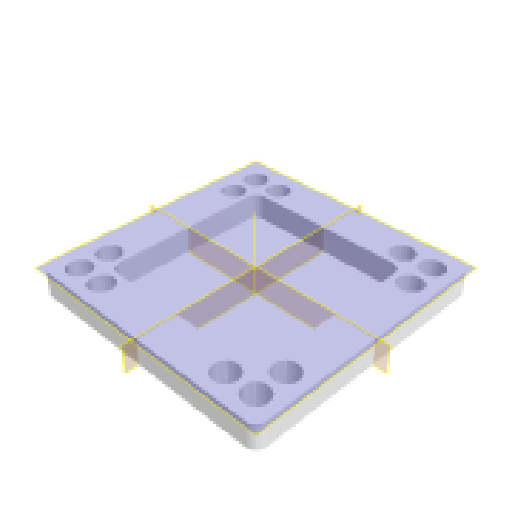
# Autodesk Inventor part: 10_Base_v4
Saved by Autodesk Inventor 2025.1 (Build 291241020, 241B)
## iProperties
Created: 2024-08-19
Part Number: 10_Base_v4
Material: Generisch
Document SubType Name: Modeling
Designer: diederichbenedict
Density: 1 g/cm^3
Appearance: Smooth - White
Author: diederichbenedict
Autodesk Inventor part; units mm, degrees
ref_plane "YZ Plane" through (0, 0, 0) normal (1, 0, 0) x (0, 1, 0)
ref_plane "XZ Plane" through (0, 0, 0) normal (0, 1, 0) x (-1, 0, 0)
ref_plane "XY Plane" through (0, 0, 0) normal (0, 0, 1) x (1, 0, 0)
ref_plane "Arbeitsebene1" through (21.5439, 0, 2.0695) normal (0, 0, -1) x (-1, 0, 0)
sketch "Skizze1" plane through (21.5439, 0, 2.0695) normal (0, 0, -1) x (-1, 0, 0)
  line L0 (-25, -25) -> (25, -25)
  line L1 (25, -25) -> (25, 25)
  line L2 (25, 25) -> (-25, 25)
  line L3 (-25, 25) -> (-25, -25)
  line L4 (-25, -25) -> (25, 25) construction
  line L5 (25, -25) -> (-25, 25) construction
  line L6 (-17, -17) -> (17, -17)
  line L7 (17, -17) -> (17, 17)
  line L8 (17, 17) -> (-17, 17)
  line L9 (-17, 17) -> (-17, -17)
  line L10 (-17, -17) -> (17, 17) construction
  line L11 (17, -17) -> (-17, 17) construction
  point P0 (21.5439, 0)
  point P1 (0, 0)
  point P2 (0, 0)
  dimension "d0" = 50
  dimension "d1" = 50
  dimension "d2" = 34
  dimension "d3" = 34
  constraints: 24 end point, 5 midpoint, 4 parallel, 2 horizontal, 2 perpendicular
  measures "d0" distance of L2.end L1.end
  measures "d1" distance of L1.end L0.end
  measures "d2" distance of L8.end L7.end
  measures "d3" distance of L7.end L6.end
extrude "Extrusion1" add sketch "Skizze1" along normal blind 5
sketch "Skizze2" plane through (21.5439, 0, -2.9305) normal (0, 0, -1) x (-1, 0, 0)
  line L0 (21, 17) -> (21, -17) projected
  line L1 (25, -25) -> (25, 25) projected
  line L2 (25, 25) -> (-25, 25) projected
  line L3 (-25, 25) -> (-25, -25) projected
  line L4 (-25, -25) -> (25, -25) projected
  line L5 (-17, -17) -> (-17, 17) projected
  line L6 (-17, 17) -> (17, 17) projected
  line L7 (17, 17) -> (17, -17) projected
  line L8 (17, -17) -> (-17, -17) projected
  line L9 (20.5, -20.5) -> (-20.5, -20.5)
  line L10 (-20.5, -20.5) -> (-20.5, 20.5)
  line L11 (-20.5, 20.5) -> (20.5, 20.5)
  line L12 (20.5, 20.5) -> (20.5, -20.5)
  line L13 (20.5, -20.5) -> (-20.5, 20.5) construction
  line L14 (-20.5, -20.5) -> (20.5, 20.5) construction
  point P0 (21.5439, 0)
  point P1 (0, 0)
  point P2 (-14.5, 20.5)
  point P3 (-20.5, 14.5)
  dimension "d6" = 41
  dimension "d7" = 41
  dimension "d_pin" = 14.5
  dimension "d10" = 14.5
  constraints: 12 end point, 2 midpoint, 2 parallel, 2 point on line, 1 horizontal, 1 perpendicular
  measures "d6" distance of L10.end L11.end
  measures "d7" distance of L9.end L10.end
  measures "d_pin" horizontal distance of point (-14.5, 20.5) point (0, 0)
  measures "d10" vertical distance of point (0, 0) point (-20.5, 14.5)
hole "Bohrung1" at (36.0439, 20.5, -2.9305) at (42.0439, 14.5, -2.9305) at (42.0439, 20.5, -2.9305) direction (0, 0, 1) diameter 4.8 end through all
ref_plane "Arbeitsebene2" through (21.5439, -25, 2.0695) normal (1, 0, 0) x (0, 0, -1)
ref_plane "Arbeitsebene3" through (-3.4561, 0, 2.0695) normal (0, -1, 0) x (1, 0, 0)
pattern_circular "Runde Anordnung1" count 4 over 360 about axis through (21.5439, 0, 2.0695) along (0, 0, 1) of "Bohrung1"
fillet "Rundung1" radius 2 8 edges at (38.5439, 17, -0.4305) (38.5439, -17, -0.4305) (4.5439, -17, -0.4305) (4.5439, 17, -0.4305) (-3.4561, 25, -0.4305) (-3.4561, -25, -0.4305) (46.5439, -25, -0.4305) (46.5439, 25, -0.4305)
equation "\"d10\" = d_pin"
